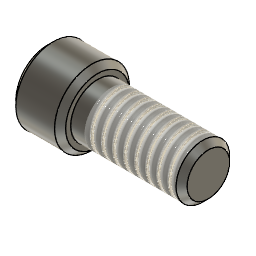
m2 bolt 4mm v1 (Autodesk Fusion 360 design; units mm, degrees)
Autodesk Fusion 360 part; units mm, degrees
sketch "Sketch1" plane through (0, 0, 0) normal (1, 0, 0) x (0, 1, 0)
  circle A0 centre (0, 0) radius 1.35
  line L0 (0, 0.866) -> (-0.75, 0.433)
  line L1 (-0.75, 0.433) -> (-0.75, -0.433)
  line L2 (-0.75, -0.433) -> (0, -0.866)
  line L3 (0, -0.866) -> (0.75, -0.433)
  line L4 (0.75, -0.433) -> (0.75, 0.433)
  line L5 (0.75, 0.433) -> (0, 0.866)
  line L6 (-0.75, -0.433) -> (0.75, 0.433) construction
  line L7 (0.75, -0.433) -> (-0.75, 0.433) construction
  line L8 (0, -0.866) -> (0, 0.866) construction
  line L9 (-0.75, -0.433) -> (0.75, -0.433) construction
  dimension "d1" = 2.7
  dimension "d2" = 1.5
  dimension "d3" = 120
  dimension "d4" = 120
  constraint coincident A0.centre origin
  constraint vertical L1
  constraint parallel L1 L4
  constraint equal L0 L5
  constraint equal L4 L5
  constraint equal L3 L4
  constraint equal L2 L3
  constraint equal L1 L2
  constraint midpoint L6 A0.centre
  measures "d1" diameter of A0
  measures "d2" horizontal distance of L1.end L3.end
  measures "d3" angle of L1 L2
  measures "d4" angle of L2 L3
extrude "Extrude1" add sketch "Sketch1" along normal blind 1.8 contours A0 | L0 L1 L2 L3 L4 L5
extrude "Extrude2" cut sketch "Sketch1" along normal blind 1 contours L0 L1 L2 L3 L4 L5
sketch "Sketch2" plane through (1.8, 0, 0) normal (1, 0, 0) x (0, 1, 0)
  circle A0 centre (0, 0) radius 1.35
  circle A1 centre (0, 0) radius 1
  dimension "d9" = 2
  constraint concentric A0 A1
  measures "d9" diameter of A1
extrude "Extrude3" add sketch "Sketch2" along normal blind 4 contours A1
thread "Thread1" "ISO Metric profile 2.0 M2x0.4 M2x0.4 6g" major diameter 1.9335 minor diameter 1.478 pitch 0.4 angle 60 resizes the face on face at (4.4667, 0.995, -0.0996) from (2.3, 0, 0) to (5.8, 0, 0)
chamfer "Chamfer1" distance 0.2 angle 45 3 edges at (0, -1.2586, -0.4882) (1.8, -1.2586, -0.4882) (5.8, -0.9013, -0.3496)
